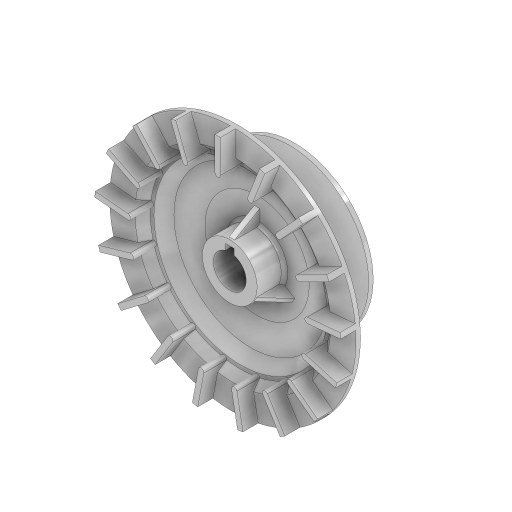
# Autodesk Inventor part: Part027. Cooling Fan
Saved by Autodesk Inventor 2023.2 (Build 272271030, 271C)
## iProperties
Created: 2023-10-07
Part Number: Part027. Cooling Fan
Material: Aluminum 6061-AHC
Document SubType Name: Modeling
Designer: User
Mass: 873.331 g
Surface Area: 1477.57 cm^2
Volume: 323.456 cm^3
Density: 2.7 g/cm^3
Appearance: Aluminum - Polished
Author: User
Autodesk Inventor part; units mm, degrees
ref_plane "YZ Plane" through (0, 0, 0) normal (1, 0, 0) x (0, 1, 0)
ref_plane "XZ Plane" through (0, 0, 0) normal (0, 1, 0) x (-1, 0, 0)
sketch "Sketch1" plane through (0, 0, 0) normal (1, 0, 0) x (0, 1, 0)
  line L0 (-72, 4.1411) -> (-39, 12.9834)
  line L1 (-39, 12.9834) -> (-39, 27.5714)
  line L2 (-39, 27.5714) -> (-72, 36.4137)
  line L3 (0, -11.8) -> (0, 70.8) projected
  line L4 (-72, 36.4137) -> (-80.7274, 45.1411)
  line L5 (-80.7274, 45.1411) -> (-84, 45.1411)
  line L6 (-84, 45.1411) -> (-91, 52.1411)
  line L7 (-91, 52.1411) -> (-112.5, 52.1411)
  line L8 (-72, 0) -> (-35, 9.9141)
  line L9 (-35, 9.9141) -> (-35, 30.6407)
  line L10 (-35, 30.6407) -> (-69.9294, 40)
  line L11 (-69.9294, 40) -> (-79.0706, 49.1411)
  line L12 (-79.0706, 49.1411) -> (-82.3431, 49.1411)
  line L13 (-82.3431, 49.1411) -> (-89.3431, 56.1411)
  line L14 (-89.3431, 56.1411) -> (-112.5, 56.1411)
  line L15 (-72, 4.1411) -> (-72, 0)
  line L16 (-112.5, 56.1411) -> (-112.5, 52.1411)
  line L17 (-15, 59) -> (-25, 59)
  line L18 (-25, 59) -> (-25, 34)
  line L19 (-25, 24) -> (-15, 24)
  line L20 (-15, 24) -> (-15, 59)
  line L21 (-25, 29) -> (-35, 29)
  line L22 (-25, 34) -> (-47.5371, 34)
  line L23 (-25, 34) -> (-25, 29) construction
  line L24 (-25, 29) -> (-25, 24)
  point P0 (0, 0)
  dimension "d0" = 30
  dimension "d1" = 78
  dimension "d2" = 135
  dimension "d3" = 45
  dimension "d4" = 41
  dimension "d5" = 48
  dimension "d6" = 144
  dimension "d7" = 182
  dimension "d8" = 4
  dimension "d9" = 40
  dimension "d10" = 225
  dimension "d11" = 70
  dimension "d12" = 30
  dimension "d13" = 50
  dimension "d14" = 35
  dimension "d15" = 24
  dimension "d16" = 5
  dimension "d17" = 10
  constraints: 48 end point, 6 perpendicular, 4 horizontal, 4 parallel, 3 point on line, 3 vertical, 1 equal length, 1 horizontal alignment, 1 vertical alignment, 5 other
  measures "d0" angle of L0 L2
  measures "d1" diameter of L1 L3
  measures "d2" angle of L5 L4
  measures "d3" angle of L7 L6
  measures "d4" distance from line of L0.start L5
  measures "d5" distance from line of L0.start L7
  measures "d6" diameter of L0.start L3
  measures "d7" diameter of L6.end L3
  measures "d8" distance between parallel lines of L0 L8
  measures "d9" vertical distance of L8.start L10.end
  measures "d10" diameter of L16 L3
  measures "d11" diameter of L9 L3
  measures "d12" diameter of L20 L3
  measures "d13" diameter of L18 L3
  measures "d14" distance of L19.end L17.start
  measures "d15" distance from line of point (0, 0) L19
  measures "d16" distance between parallel lines of L19 L21
  measures "d17" distance between parallel lines of L19 L22
revolve "Revolution1" add sketch "Sketch1" angle 360 about axis through (0, 0, -10) along (0, 0, 1)
fillet "Fillet1" radius 3 3 edges at (0, 25, 34) (0, 35, 29) (0, 25, 29)
fillet "Fillet1" radius 6 2 edges at (0, 39, 27.5714) (0, 39, 12.9834)
fillet "Fillet1" radius 10 1 edges at (0, 35, 9.9141)
ref_plane "Work Plane1" through (0, 0, 70) normal (0, 0, 1) x (1, 0, 0)
sketch "Sketch2" plane through (0, 0, 70) normal (0, 0, 1) x (1, 0, 0)
  line L0 (-2.5, 112.4722) -> (-2.5, 82.5)
  arc A0 (-2.5, 82.5) -> (2.5, 82.5) centre (0, 82.5) ccw
  line L1 (2.5, 82.5) -> (2.5, 112.4722)
  circle A1 centre (0, 0) radius 112.5 projected
  arc A2 (2.5, 112.4722) -> (-2.5, 112.4722) centre (0, 0) ccw
  dimension "d23" = 5
  dimension "d24" = 32.5
  constraints: 6 point on circle, 4 end point, 2 centre point, 2 tangent, 1 parallel, 1 vertical, 1 vertical alignment
  measures "d23" distance between parallel lines of L1 L0
extrude "Extrusion1" add sketch "Sketch2" against normal up to next contours A1 L1 A0 L0 picked at (0.2778, 92.499)
pattern_circular "Circular Pattern1" count 17 over 360 about axis through (0, 0, 54.1411) along (0, 0, 1) of "Extrusion1"
sketch "Sketch3" plane through (0, 0, 0) normal (1, 0, 0) x (0, 1, 0)
  line L0 (25, 57) -> (36.4935, 37.0928)
  line L1 (25, 37) -> (25, 59) construction
  line L2 (0, -14) -> (0, 84) construction
  line L3 (25, 59) -> (-25, 59) projected
  point P0 (0, 0)
  dimension "d30" = 30
  dimension "d31" = 2
  constraints: 2 end point, 1 point on line
  measures "d30" angle of L2 L0
  measures "d31" distance from line of L3 L0.start
extrude "Rib1" add sketch "Sketch3" along normal mid plane 5 rib yes fills toward (30.7034, 47.0214) open curves L0
pattern_circular "Circular Pattern2" count 3 over 360 about axis through (0, 0, 46.5) along (0, 0, 1) of "Rib1"
sketch "Sketch4" plane through (0, 0, 59) normal (0, 0, 1) x (1, 0, 0)
  circle A0 centre (0, 0) radius 15 projected
  line L0 (-4, 20) -> (4, 20)
  line L1 (4, 20) -> (4, 0)
  line L2 (4, 0) -> (-4, 0)
  line L3 (-4, 0) -> (-4, 20)
  dimension "d41" = 20
  dimension "d42" = 8
  constraints: 8 end point, 2 parallel, 1 coincident, 1 horizontal, 1 midpoint, 1 perpendicular
  measures "d41" distance from line of A0.centre L0
  measures "d42" distance between parallel lines of L1 L3
extrude "Extrusion2" cut sketch "Sketch4" against normal through all contours L1 L2 L3 A0 | A0 L3 L0 L1 picked at (0.4493, 4.9798)
body "Solid1"
